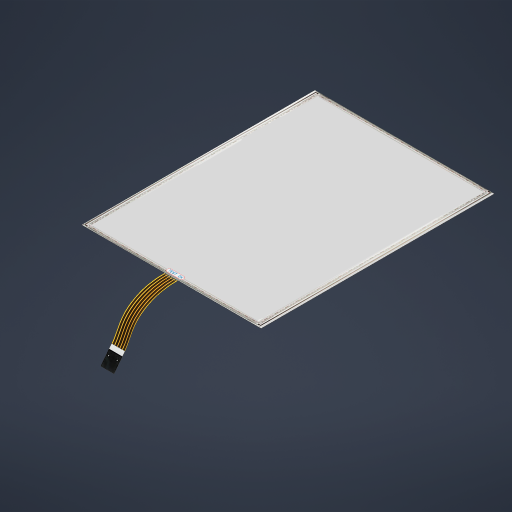
# Autodesk Inventor part: 12inch Touchscreen
Saved by Autodesk Inventor 2023 (Build 270158000, 158)
## iProperties
Created: 2023-02-24
Part Number: 12inch Touchscreen
Material: Generic
Document SubType Name: Modeling
Designer: roota
Density: 1 g/cm^3
Appearance: Default
Author: roota
Autodesk Inventor part; units mm, degrees
ref_plane "YZ Plane" through (0, 0, 0) normal (1, 0, 0) x (0, 1, 0)
ref_plane "XZ Plane" through (0, 0, 0) normal (0, 1, 0) x (-1, 0, 0)
ref_plane "XY Plane" through (0, 0, 0) normal (0, 0, 1) x (1, 0, 0)
sketch "Sketch1" plane through (0, 0, 0) normal (0, 1, 0) x (-1, 0, 0)
  line L0 (100, 130) -> (-100, 130)
  line L1 (-100, 130) -> (-100, -130)
  line L2 (-100, -130) -> (100, -130)
  line L3 (100, -130) -> (100, 130)
  line L4 (100, 130) -> (-100, -130) construction
  line L5 (-100, 130) -> (100, -130) construction
  point P0 (0, 0)
  dimension "d0" = 200
  dimension "d1" = 260
  constraints: 12 end point, 2 midpoint, 2 parallel, 1 horizontal, 1 perpendicular
  measures "d0" distance of L2.end L1.end
  measures "d1" distance of L1.end L0.end
extrude "Extrusion1" add sketch "Sketch1" along normal blind 0.188
sketch "Sketch2" plane through (0, 0, 0) normal (1, 0, 0) x (0, 1, 0)
  line L0 (0.188, 130) -> (0.188, -130) projected
  line L1 (0, 90.3171) -> (0, 130) construction
  spline S0 degree 4 poles (0, 130) (0, 139.6494) (-1.5898, 157.4531) (-13.2721, 180.5855) (-31.4832, 183.4994) (-38.5468, 188.9997) knots 0 0 0 0 0 0.504551 1 1 1 1 1
  line L2 (0, 130) -> (0, 216.7) construction
  line L3 (-38.5468, 188.9997) -> (-50.3819, 198.2154) construction
  point P0 (0, 0)
  point P1 (-3.8232, 155.3879)
  point P2 (-18.7307, 177.3655)
  dimension "d4" = 86.7
  dimension "d10" = 15
  constraints: 6 end point, 3 vertical, 1 coincident, 5 other
  measures "d4" distance of L1.end L2.end
  measures "d10" distance of L3.start L3.end
sketch "Sketch3" plane through (0, 0, 0) normal (1, 0, 0) x (0, 1, 0)
  spline S0 degree 4 poles (0, 130) (0, 139.6494) (-1.5898, 157.4531) (-13.2721, 180.5855) (-31.4832, 183.4994) (-38.5468, 188.9997) knots 0 0 0 0 0 0.504551 1 1 1 1 1 projected
  line L0 (-38.4853, 189.0786) -> (-38.5468, 188.9997)
  line L1 (0, 130) -> (0, -130) projected
  line L2 (0, 130) -> (0.1, 130)
  line L3 (0, 130) -> (0.188, 130) projected
  spline S1 degree 5 poles (0.1, 130) (0.0999, 132.5176) (0.0491, 135.0352) (-0.0819, 137.5517) (-0.551, 142.6368) (-1.4697, 147.6604) (-2.0608, 150.1807) (-3.5179, 155.2385) (-5.5009, 160.1155) (-6.6465, 162.5358) (-9.1757, 167.1539) (-12.3042, 171.387) (-14.0003, 173.3478) (-17.6139, 176.8534) (-21.7361, 179.7401) (-23.8355, 180.9926) (-28.0959, 183.233) (-32.4319, 185.3278) (-34.5534, 186.3923) (-36.6108, 187.6177) (-38.4853, 189.0786) knots 0 0 0 0 0 0 0.16598 0.16598 0.16598 0.336346 0.336346 0.336346 0.512543 0.512543 0.512543 0.682634 0.682634 0.682634 0.843325 0.843325 0.843325 1 1 1 1 1 1
  point P0 (0, 0)
  dimension "d5" = 0.1
  constraints: 4 end point, 1 collinear, 4 other
extrude "Extrusion2" add sketch "Sketch3" along normal mid plane 15
sketch "Sketch4" plane through (-7.5, -38.5468, 188.9997) normal (0, -0.7890077, 0.6143833) x (1, 0, 0)
  line L0 (0, 0) -> (0, 0.1) projected
  line L1 (0, 0.1) -> (15, 0.1) projected
  line L2 (0, 0) -> (15, 0)
  line L3 (15, 0) -> (15, 0.1)
  line L4 (15, 0.1) -> (0, 0.1)
  line L5 (0, 0.1) -> (0, 0)
  point P0 (7.5, -125.4397)
  constraints: 8 end point, 2 parallel, 1 horizontal, 1 perpendicular
extrude "Extrusion3" add sketch "Sketch4" along normal blind 20
sketch "Sketch5" plane through (0, 0.188, 0) normal (0, 1, 0) x (1, 0, 0)
  line L0 (-7.5, -226.5029) -> (-7.5, -130) construction
  line L1 (-7.5, -130) -> (7.5, -130) construction
  line L2 (7.5, -130) -> (7.5, -226.5029) construction
  line L3 (7.5, -226.5029) -> (-7.5, -226.5029) construction
  point P0 (0, 0)
  constraints: 2 coincident, 2 other
decal "Decal1"
sketch "Sketch6" plane through (-7.5, -38.4853, 189.0786) normal (0, 0.6143833, 0.7890077) x (1, 0, 0)
  line L0 (0.0146, -20.011) -> (0, 0) construction
  line L1 (0, 0) -> (14.9854, 0.011) construction
  line L2 (14.9854, 0.011) -> (15, -20) construction
  line L3 (15, -20) -> (0.0146, -20.011) construction
  point P0 (7.5, 146.5319)
  constraints: 2 coincident, 2 other
decal "Decal2"
sketch "Sketch7" plane through (7.5, -38.5468, 188.9997) normal (0, -0.6143833, -0.7890077) x (-1, 0, 0)
  line L0 (0.0146, -20.011) -> (0, 0) construction
  line L1 (0, 0) -> (14.9854, 0.011) construction
  line L2 (14.9854, 0.011) -> (15, -20) construction
  line L3 (15, -20) -> (0.0146, -20.011) construction
  point P0 (7.5, 146.5319)
  constraints: 2 coincident, 2 other
decal "Decal3"
sketch "Sketch8" plane through (0, 0, 0) normal (0, -1, 0) x (1, 0, 0)
  line L0 (7.5, 207.6879) -> (7.5, 130) construction
  line L1 (7.5, 130) -> (-7.5, 130) construction
  line L2 (-7.5, 130) -> (-7.5, 207.6879) construction
  line L3 (-7.5, 207.6879) -> (7.5, 207.6879) construction
  point P0 (0, 0)
  constraints: 2 coincident, 2 other
decal "Decal4"
sketch "Sketch10" plane through (0, 0.188, 0) normal (0, 1, 0) x (1, 0, 0)
  line L0 (98.0274, 130) -> (98.0274, -130) construction
  line L1 (98.0274, -130) -> (-100, -130) construction
  line L2 (-100, -130) -> (-100, 130) construction
  line L3 (-100, 130) -> (98.0274, 130) construction
  point P0 (0, 0)
  constraints: 2 coincident, 2 other
decal "Decal6"
sketch "Sketch11" plane through (0, 0, 0) normal (0, -1, 0) x (1, 0, 0)
  line L0 (-98.7516, -130.9508) -> (-100, 130) construction
  line L1 (-100, 130) -> (98.7516, 130.9508) construction
  line L2 (98.7516, 130.9508) -> (100, -130) construction
  line L3 (100, -130) -> (-98.7516, -130.9508) construction
  point P0 (0, 0)
  constraints: 2 coincident, 2 other
decal "Decal7"
sketch "Sketch9" plane through (0, 0.188, 0) normal (0, 1, 0) x (1, 0, 0)
  line L0 (-9.9844, -128.5553) -> (-9.9844, -122.1467) construction
  line L1 (-9.9844, -122.1467) -> (9.7409, -122.1467) construction
  line L2 (9.7409, -122.1467) -> (9.7409, -128.5553) construction
  line L3 (9.7409, -128.5553) -> (-9.9844, -128.5553) construction
  point P0 (0, 0)
  constraints: 2 other
decal "Decal5"
body "Solid1"
